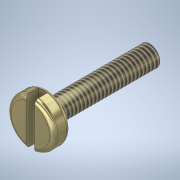
# Autodesk Inventor part: ScrewM3x12
Saved by Autodesk Inventor 2020 (Build 240168000, 168)
## iProperties
Created: 2018-12-27
Part Number: ScrewM3x12
Material: Stainless Steel
Document SubType Name: Modeling
Designer: Victor Sabino
Density: 8 g/cm^3
Appearance: Semi-Polished
Mass: 0.604027 g
Surface Area: 1.55601 cm^2
Volume: 0.0755034 cm^3
Author: Victor Sabino
Autodesk Inventor part; units mm, degrees
ref_plane "YZ Plane" through (0, 0, 0) normal (1, 0, 0) x (0, 1, 0)
ref_plane "XZ Plane" through (0, 0, 0) normal (0, 1, 0) x (-1, 0, 0)
ref_plane "XY Plane" through (0, 0, 0) normal (0, 0, 1) x (1, 0, 0)
sketch "Sketch1" plane through (0, 0, 0) normal (0, 0, 1) x (1, 0, 0)
  circle A0 centre (0, 0) radius 2.75
  dimension "d0" = 5.5
  constraints: 1 centre point, 1 coincident
  measures "d0" diameter of A0
extrude "Extrusion1" add sketch "Sketch1" against normal blind 2
sketch "Sketch2" plane through (0, 0, 0) normal (0, 0, 1) x (1, 0, 0)
  line L0 (-0.5, 2.75) -> (0.5, 2.75)
  line L1 (0.5, 2.75) -> (0.5, -2.75)
  line L2 (0.5, -2.75) -> (-0.5, -2.75)
  line L3 (-0.5, -2.75) -> (-0.5, 2.75)
  line L4 (-0.5, 2.75) -> (0.5, -2.75) construction
  line L5 (0.5, 2.75) -> (-0.5, -2.75) construction
  point P0 (0, 0)
  dimension "d3" = 1
  dimension "d4" = 5.5
  constraints: 12 end point, 2 midpoint, 2 parallel, 1 horizontal, 1 perpendicular
  measures "d3" distance of L1.end L2.end
  measures "d4" distance of L0.end L1.end
extrude "Extrusion2" cut sketch "Sketch2" against normal blind 1.5
sketch "Sketch3" plane through (0, 0, -2) normal (0, 0, -1) x (-1, 0, 0)
  circle A0 centre (0, 0) radius 1.2
  dimension "d7" = 2.4
  constraints: 1 centre point, 1 coincident
  measures "d7" diameter of A0
extrude "Extrusion3" add sketch "Sketch3" along normal blind 12
thread "Thread2" size "M2.5x0.45" class "6g" standard "ANSI Metric M Profile" full length
fillet "Fillet1" radius 0.5 5 edges at (1.2, 0, -2) (-2.75, 0, -2) (-2.75, 0, 0) (2.1139, 1.7589, 0) (2.1139, -1.7589, 0)
body "Solid1"
